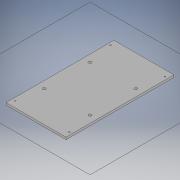
# Autodesk Inventor part: 000.001.006 - Площадка под манипулятор
Saved by Autodesk Inventor 2022 (Build 260153000, 153)
## iProperties
Created: 2022-02-27
Part Number: 000.001.006 - Площадка под манипулятор
Material: Типовые
Document SubType Name: Modeling
Designer: Petrov Ivan
Density: 1 g/cm^3
Appearance: По умолчанию
Author: Petrov Ivan
Autodesk Inventor part; units mm, degrees
ref_plane "YZ Plane" through (0, 0, 0) normal (1, 0, 0) x (0, 1, 0)
ref_plane "XZ Plane" through (0, 0, 0) normal (0, 1, 0) x (-1, 0, 0)
ref_plane "XY Plane" through (0, 0, 0) normal (0, 0, 1) x (1, 0, 0)
sketch "Эскиз1" plane through (0, 0, 0) normal (0, 1, 0) x (-1, 0, 0)
  line L0 (-80, 144) -> (80, 144)
  line L1 (80, 144) -> (80, -144)
  line L2 (80, -144) -> (-80, -144)
  line L3 (-80, -144) -> (-80, 144)
  line L4 (-80, 144) -> (80, -144) construction
  line L5 (80, 144) -> (-80, -144) construction
  point P0 (0, 0)
  dimension "d0" = 160
  dimension "d1" = 288
  constraints: 12 end point, 2 midpoint, 2 parallel, 1 horizontal, 1 perpendicular
  measures "d0" distance of L1.end L2.end
  measures "d1" distance of L0.end L1.end
extrude "Выдавливание1" add sketch "Эскиз1" along normal blind 6
sketch "Эскиз2" plane through (0, 0, 0) normal (0, -1, 0) x (1, 0, 0)
  circle A0 centre (-72.875, -128) radius 2 projected
  circle A1 centre (72, -128) radius 1.85 projected
  circle A2 centre (72.875, 128) radius 2 projected
  circle A3 centre (-72, 128) radius 1.85 projected
  point P0 (0, 0)
extrude "Выдавливание2" cut sketch "Эскиз2" against normal through all
sketch "Эскиз3" plane through (0, 0, 0) normal (0, -1, 0) x (1, 0, 0)
  circle A0 centre (-61.2572, -61.2572) radius 4 projected
  circle A1 centre (-61.2572, 61.2572) radius 4 projected
  circle A2 centre (61.2572, 61.2572) radius 4 projected
  circle A3 centre (61.2572, -61.2572) radius 4 projected
  point P0 (0, 0)
extrude "Выдавливание3" cut sketch "Эскиз3" against normal through all
